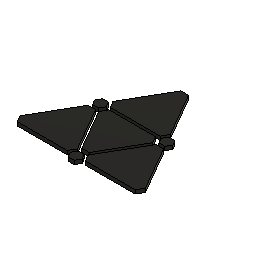
FumeExtractorFusionCAD (Autodesk Fusion 360 archive; units mm, degrees)
design "logoV2"
Autodesk Fusion 360 part; units mm, degrees
sketch "Sketch1" plane through (0, 0, 0) normal (0, 0, 1) x (1, 0, 0)
  line L0 (-18.1865, -0.75) -> (-35.507, -30.75)
  line L1 (-35.507, -30.75) -> (-0.866, -30.75)
  line L2 (-0.866, -30.75) -> (-18.1865, -0.75)
  line L3 (17.3205, 0.75) -> (0, 30.75)
  line L4 (-17.3205, 0.75) -> (17.3205, 0.75)
  line L5 (0, 30.75) -> (-17.3205, 0.75)
  line L6 (35.507, -30.75) -> (18.1865, -0.75)
  line L7 (0.866, -30.75) -> (35.507, -30.75)
  line L8 (18.1865, -0.75) -> (0.866, -30.75)
  line L9 (0, 10.75) -> (0, 0.75) construction
  line L10 (-17.3205, 0.75) -> (-18.1865, -0.75) construction
  line L11 (17.3205, 0.75) -> (18.1865, -0.75) construction
  line L12 (16.4545, -0.75) -> (0, -29.25)
  line L13 (-16.4545, -0.75) -> (16.4545, -0.75)
  line L14 (0, -29.25) -> (-16.4545, -0.75)
  point P0 (-18.1865, -20.75)
  point P1 (0, 10.75)
  point P2 (18.1865, -20.75)
  dimension "d2" = 10
  dimension "d3" = 10
  dimension "d4" = 10
  dimension "d6" = 34.641
  dimension "d8" = 20
  dimension "d9" = 20.75
  dimension "d11" = 0.75
  dimension "d16" = 1.5
  dimension "d17" = 1.5
  dimension "d18" = 1.5
  constraint horizontal L1
  constraint horizontal L4
  constraint horizontal L7
  constraint horizontal P0 P2
  constraint coincident P1 L9.start
  constraint vertical L9
  constraint coincident L4 L9.end
  constraint vertical origin L9.end
  constraint parallel L5 L10
  constraint coincident L0.start L2.end
  constraint parallel L3 L11
  constraint coincident L6.end L8.start
  constraint coincident L13.start L14.end
  constraint coincident L12.start L13.end
  constraint coincident L12.end L14.start
  measures "d2" distance of P0 L2
  measures "d3" distance of P1 L3
  measures "d4" distance of P2 L6
  measures "d6" distance of L0.end L1.end
  measures "d8" distance of L0.start P0
  measures "d9" vertical distance of origin P0
  measures "d11" distance of origin L9.end
extrude "Extrude1" add sketch "Sketch1" along normal blind 2 makes body 1 at (0, 10.75, 0) makes body 2 at (-18.1865, -20.75, 0) makes body 3 at (18.1865, -20.75, 0) makes body 4 at (0, -10.25, 0)
chamfer "Chamfer1" distance 4 angle 45 9 edges at (0.866, -30.75, 1) (35.507, -30.75, 1) (18.1865, -0.75, 1) (-0.866, -30.75, 1) (-35.507, -30.75, 1) (-18.1865, -0.75, 1) (17.3205, 0.75, 1) (0, 30.75, 1) (-17.3205, 0.75, 1) on bodies 1 2 3
chamfer "Chamfer2" distance 4 angle 45 3 edges at (0, -29.25, 1) (16.4545, -0.75, 1) (-16.4545, -0.75, 1) on bodies 4
sketch "Sketch2" plane through (0, 0, 2) normal (0, 0, 1) x (-1, 0, 0)
  line L0 (12.4545, 0.75) -> (14.4545, 4.2141)
  line L1 (14.4545, 4.2141) -> (2, 25.7859)
  line L2 (2, 25.7859) -> (-2, 25.7859)
  line L3 (-2, 25.7859) -> (-14.4545, 4.2141)
  line L4 (-14.4545, 4.2141) -> (-12.4545, 0.75)
  line L5 (-12.4545, 0.75) -> (12.4545, 0.75)
  line L6 (16.1865, 4.2141) -> (20.1865, 4.2141)
  line L7 (20.1865, 4.2141) -> (33.507, 27.2859)
  line L8 (33.507, 27.2859) -> (31.507, 30.75)
  line L9 (31.507, 30.75) -> (4.866, 30.75)
  line L10 (4.866, 30.75) -> (2.866, 27.2859)
  line L11 (2.866, 27.2859) -> (16.1865, 4.2141)
  line L12 (-20.1865, 4.2141) -> (-16.1865, 4.2141)
  line L13 (-16.1865, 4.2141) -> (-2.866, 27.2859)
  line L14 (-2.866, 27.2859) -> (-4.866, 30.75)
  line L15 (-4.866, 30.75) -> (-31.507, 30.75)
  line L16 (-31.507, 30.75) -> (-33.507, 27.2859)
  line L17 (-33.507, 27.2859) -> (-20.1865, 4.2141)
  line L18 (4.866, 30.75) -> (-4.866, 30.75)
  line L19 (2.433, 26.5359) -> (4.866, 30.75)
  line L20 (4.866, 30.75) -> (2.433, 34.9641)
  line L21 (2.433, 34.9641) -> (-2.433, 34.9641)
  line L22 (-2.433, 34.9641) -> (-4.866, 30.75)
  line L23 (-4.866, 30.75) -> (-2.433, 26.5359)
  line L24 (-2.433, 26.5359) -> (2.433, 26.5359)
  line L25 (1.567, 28.0359) -> (3.134, 30.75)
  line L26 (3.134, 30.75) -> (1.567, 33.4641)
  line L27 (1.567, 33.4641) -> (-1.567, 33.4641)
  line L28 (-1.567, 33.4641) -> (-3.134, 30.75)
  line L29 (-3.134, 30.75) -> (-1.567, 28.0359)
  line L30 (-1.567, 28.0359) -> (1.567, 28.0359)
  line L31 (0, 25.7859) -> (0, 0.75) construction
  line L32 (8.2272, 15) -> (-13.4545, 2.4821) construction
  line L33 (-8.2272, 15) -> (13.4545, 2.4821) construction
  point P0 (0, 30.75)
  point P1 (0, 30.75)
  point P2 (0, 10.25)
  dimension "d20" = 1.5
  constraint coincident L9.end L10.start
  constraint coincident L14.end L15.start
  constraint midpoint L18 P1
  constraint horizontal L24
  constraint coincident L10.end L19
  constraint coincident P1 P0
  constraint midpoint L2 L31.start
  constraint midpoint L5 L31.end
  constraint midpoint L1 L32.start
  constraint midpoint L4 L32.end
  constraint midpoint L3 L33.start
  constraint midpoint L0 L33.end
  constraint coincident L31 P2
  constraint coincident L33 P2
  measures "d20" distance of L24 L30
extrude "Extrude2" add sketch "Sketch2" against normal blind 2 separate body contours L18 L25 L29 L30 | L18 L26 L27 L28 makes body 5
pattern_circular "C-Pattern1" count 3 over 360 about axis through (0, -10.25, -128.8735) along (0, 0, 1) of "Extrude2" makes body 6 at (18.7982, 0, 2) makes body 7 at (-16.7089, 0, 2)
equation "scale = 1 mm"
equation "d2 = 10 * scale"
equation "d3 = d2"
equation "d4 = d2"
equation "d5 = d6 / 2 + spacing / 2"
equation "d9 = d8 + spacing / 2"
equation "spacing = 1.5 * scale"
equation "d11 = spacing / 2"
equation "d12 = height"
equation "d14 = chamfer"
equation "chamfer = 4 * scale"
equation "d16 = spacing"
equation "d17 = spacing"
equation "d18 = spacing"
equation "d19 = chamfer"
equation "d20 = spacing"
equation "d21 = -height"
equation "height = 2 mm"

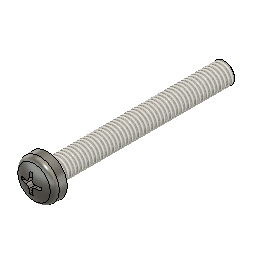
design "Pan Head Screw ISO 7045 - M3 x 25 - H Steel 4.6 Plain"
description: Pan Head Screw ISO 7045 - M3 x 25 - H
part number: ISO 7045 - M3 x 25 - H Steel 4.6 Plain
Autodesk Fusion 360 part; units mm, degrees
sketch "Sketch1" plane through (0, 0, 0) normal (0, 1, 0) x (1, 0, 0)
  line L0 (-1.5, 1) -> (-1.5, 25)
  line L1 (-1.5, 25) -> (0, 25)
  line L2 (0, 25) -> (0, -2.4)
  line L3 (-1.3647, 0) -> (-2.8, 0)
  arc A0 (-2.7449, -1.5792) -> (0, -2.4) centre (0, 2.6) ccw
  line L4 (-1.5, 1) -> (-1.3647, 0.7098)
  line L5 (-1.3647, 0.7098) -> (-1.3647, 0)
  line L6 (-2.8, 0) -> (-2.7449, -1.5792)
  dimension "d9" = 3
  dimension "d66" = 5.6
  dimension "d75" = 2.7294
  dimension "d77" = 1
  dimension "d78" = 155
  dimension "d103" = 2
  dimension "d111" = 2.4
  dimension "d112" = 25
  constraint perpendicular L0 L1
  constraint collinear origin L2.end L1.end
  constraint perpendicular L0 L3
  constraint coincident origin L3
  constraint vertical L0
  constraint vertical L2
  constraint coincident L2 A0.centre
  constraint perpendicular L3 L5
  constraint coincident L3.start L5.end
  measures "d77" distance of L3 L0.start
  measures "d78" angle of L0 L4
  measures "d103" angle of L2 L6
  measures "d111" distance of L2.end L3
  measures "d112" distance of origin L1
revolve "Revolve1" add sketch "Sketch1" angle 360 about axis through (0, 0, -25) along (0, 0, 1) makes body 1
ref_plane "WorkPlane1" through (0, 0, 2.4) normal (0, 0, 1) x (1, 0, 0)
sketch "Sketch2" plane through (0, 0, 2.4) normal (0, 0, 1) x (1, 0, 0)
  line L0 (-0.215, 0.215) -> (-1.5, 0.215)
  line L1 (-0.215, -0.215) -> (-1.5, -0.215)
  line L2 (-1.5, 0.215) -> (-1.5, -0.215)
  line L3 (-0.215, -0.215) -> (-0.215, -1.5)
  line L4 (-0.215, -1.5) -> (0.215, -1.5)
  line L5 (0.215, -0.215) -> (0.215, -1.5)
  line L6 (0.215, -0.215) -> (1.5, -0.215)
  line L7 (1.5, -0.215) -> (1.5, 0.215)
  line L8 (0.215, 0.215) -> (1.5, 0.215)
  line L9 (0.215, 0.215) -> (0.215, 1.5)
  line L10 (0.215, 1.5) -> (-0.215, 1.5)
  line L11 (-0.215, 0.215) -> (-0.215, 1.5)
  dimension "d105" = 0.43
  dimension "d107" = 360
  dimension "d108" = 3
  constraint perpendicular L1 L2
  constraint vertical L0.start L1.start
  constraint horizontal L1
  constraint coincident L8.start L9.start
  measures "d105" distance of L0 L1
  measures "d108" distance of L2 L7
extrude "Extrude1" add sketch "Sketch2" against normal blind 1.8 draft -4 separate body makes body 2
draft "Draft1" angle -30 neutral plane through (0, 0, 2.4) pull (0, 0, 1) 4 faces at (-1.458, -0.0297, 1.8) (0.0297, -1.458, 1.8) (1.458, 0.0297, 1.8) (-0.0297, 1.458, 1.8) on bodies 2
fillet "Fillet3" radius 0.43 4 edges at (0.1521, 0.1521, 1.5) (-0.1521, 0.1521, 1.5) (0.1521, -0.1521, 1.5) (-0.1521, -0.1521, 1.5) on bodies 2
combine "Combine1" operation cut target body 1 tool bodies 2
fillet "Fillet4" radius 0.9 1 edges at (-2.5591, 0.9926, 1.5792) on bodies 1
thread "Thread1" "ISO Metric profile 3.0 M3x0.5 M3x0.5 6g" major diameter 2.927 minor diameter 2.3555 pitch 0.5 angle 60 resizes the face on face at (-1.4981, 0.0748, -9) on bodies 1
fillet "Fillet5" radius 0.3 1 edges at (-1.2723, 0.4935, 0) on bodies 1
sketch "Sketch5" plane through (0, 0, 0) normal (0, 1, 0) x (1, 0, 0)
  line L0 (-1.53, 25) -> (-1.53, 24.6933)
  line L1 (-1.53, 24.6933) -> (-1.1933, 25)
  line L2 (0, 25) -> (0, -2.4)
  line L3 (-1.53, 25) -> (0, 25)
  dimension "d114" = 0.3067
  dimension "d115" = 1.53
  dimension "d116" = 0.3367
  constraint coincident L2.start L3.end
  constraint perpendicular L2 L3
  constraint coincident L1.end L3
  constraint perpendicular L0 L3
  measures "d114" distance of L0.end L3
  measures "d115" distance of L0 L2.start
  measures "d116" distance of L0 L1.end
revolve "Revolve2" cut sketch "Sketch5" angle 360 about axis through (0, 0, -25) along (0, 0, 1) bodies 1
equation "d9 = adsk_nomdia"
equation "adsk_nomlen = 25.00 mm"
equation "adsk_headh = 2.40 mm"
equation "adsk_headdia = 5.60 mm"
equation "adsk_nomdia = 3.00 mm"
equation "adsk_phildia = 3.00 mm"
equation "d31 = -adsk_phildepth"
equation "adsk_philwidth = 0.43 mm"
equation "adsk_phildepth = 1.80 mm"
equation "d66 = adsk_headdia"
equation "d71 = adsk_headh"
equation "adsk_thrlen = 24.00 mm"
equation "d75 = adsk_shnkdia"
equation "adsk_shnkdia = 2.72937 mm"
equation "d77 = adsk_nomlen - adsk_thrlen"
equation "adsk_endpointdia = 2.38655 mm"
equation "adsk_startlen = 0.306725 mm"
equation "adsk_ovalrad = 5.00 mm"
equation "adsk_headtoprad = adsk_nomdia * 0.3"
equation "adsk_midfillet = adsk_nomdia * 0.1"
equation "d98 = adsk_midfillet"
equation "adsk_headang = 2.00 deg"
equation "d102 = adsk_headtoprad"
equation "d103 = adsk_headang"
equation "d105 = adsk_philwidth"
equation "d108 = adsk_phildia"
equation "d110 = adsk_philwidth"
equation "d111 = adsk_headh"
equation "d112 = adsk_nomlen"
equation "d113 = ( adsk_nomlen + adsk_headh ) - ( adsk_ovalrad )"
equation "d114 = adsk_startlen"
equation "d115 = adsk_nomdia * 0.51"
equation "d116 = ( adsk_nomdia * 0.51 ) - ( adsk_endpointdia / 2 )"

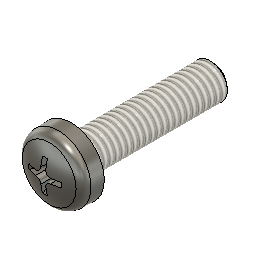
design "Pan Head Screw ISO 7045 - M3 x 12 - H Steel 4.6 Plain"
description: Pan Head Screw ISO 7045 - M3 x 12 - H
part number: ISO 7045 - M3 x 12 - H Steel 4.6 Plain
Autodesk Fusion 360 part; units mm, degrees
sketch "Sketch1" plane through (0, 0, 0) normal (0, 1, 0) x (1, 0, 0)
  line L0 (-1.5, 1) -> (-1.5, 12)
  line L1 (-1.5, 12) -> (0, 12)
  line L2 (0, 12) -> (0, -2.4)
  line L3 (-1.3647, 0) -> (-2.8, 0)
  arc A0 (-2.7449, -1.5792) -> (0, -2.4) centre (0, 2.6) ccw
  line L4 (-1.5, 1) -> (-1.3647, 0.7098)
  line L5 (-1.3647, 0.7098) -> (-1.3647, 0)
  line L6 (-2.8, 0) -> (-2.7449, -1.5792)
  dimension "d9" = 3
  dimension "d66" = 5.6
  dimension "d75" = 2.7294
  dimension "d77" = 1
  dimension "d78" = 155
  dimension "d103" = 2
  dimension "d111" = 2.4
  dimension "d112" = 12
  constraint perpendicular L0 L1
  constraint collinear origin L2.end L1.end
  constraint perpendicular L0 L3
  constraint coincident origin L3
  constraint vertical L0
  constraint vertical L2
  constraint coincident L2 A0.centre
  constraint perpendicular L3 L5
  constraint coincident L3.start L5.end
  measures "d77" distance of L3 L0.start
  measures "d78" angle of L0 L4
  measures "d103" angle of L2 L6
  measures "d111" distance of L2.end L3
  measures "d112" distance of origin L1
revolve "Revolve1" add sketch "Sketch1" angle 360 about axis through (0, 0, -12) along (0, 0, 1) makes body 1
ref_plane "WorkPlane1" through (0, 0, 2.4) normal (0, 0, 1) x (1, 0, 0)
sketch "Sketch2" plane through (0, 0, 2.4) normal (0, 0, 1) x (1, 0, 0)
  line L0 (-0.215, 0.215) -> (-1.5, 0.215)
  line L1 (-0.215, -0.215) -> (-1.5, -0.215)
  line L2 (-1.5, 0.215) -> (-1.5, -0.215)
  line L3 (-0.215, -0.215) -> (-0.215, -1.5)
  line L4 (-0.215, -1.5) -> (0.215, -1.5)
  line L5 (0.215, -0.215) -> (0.215, -1.5)
  line L6 (0.215, -0.215) -> (1.5, -0.215)
  line L7 (1.5, -0.215) -> (1.5, 0.215)
  line L8 (0.215, 0.215) -> (1.5, 0.215)
  line L9 (0.215, 0.215) -> (0.215, 1.5)
  line L10 (0.215, 1.5) -> (-0.215, 1.5)
  line L11 (-0.215, 0.215) -> (-0.215, 1.5)
  dimension "d105" = 0.43
  dimension "d107" = 360
  dimension "d108" = 3
  constraint perpendicular L1 L2
  constraint vertical L0.start L1.start
  constraint horizontal L1
  constraint coincident L8.start L9.start
  measures "d105" distance of L0 L1
  measures "d108" distance of L2 L7
extrude "Extrude1" add sketch "Sketch2" against normal blind 1.8 draft -4 separate body makes body 2
draft "Draft1" angle -30 neutral plane through (0, 0, 2.4) pull (0, 0, 1) 4 faces at (-1.458, 0.0297, 1.8) (-0.0297, -1.458, 1.8) (1.458, -0.0297, 1.8) (-0.0297, 1.458, 1.8) on bodies 2
fillet "Fillet3" radius 0.43 4 edges at (0.1521, 0.1521, 1.5) (-0.1521, 0.1521, 1.5) (0.1521, -0.1521, 1.5) (-0.1521, -0.1521, 1.5) on bodies 2
combine "Combine1" operation cut target body 1 tool bodies 2
fillet "Fillet4" radius 0.9 1 edges at (-2.5591, 0.9926, 1.5792) on bodies 1
thread "Thread1" "ISO Metric profile 3.0 M3x0.5 M3x0.5 6g" major diameter 2.927 minor diameter 2.3555 pitch 0.5 angle 60 resizes the face on face at (-1.4981, 0.0748, -4.6667) on bodies 1
fillet "Fillet5" radius 0.3 1 edges at (-1.2723, 0.4935, 0) on bodies 1
sketch "Sketch5" plane through (0, 0, 0) normal (0, 1, 0) x (1, 0, 0)
  line L0 (-1.53, 12) -> (-1.53, 11.6933)
  line L1 (-1.53, 11.6933) -> (-1.1933, 12)
  line L2 (0, 12) -> (0, -2.4)
  line L3 (-1.53, 12) -> (0, 12)
  dimension "d114" = 0.3067
  dimension "d115" = 1.53
  dimension "d116" = 0.3367
  constraint coincident L2.start L3.end
  constraint perpendicular L2 L3
  constraint coincident L1.end L3
  constraint perpendicular L0 L3
  measures "d114" distance of L0.end L3
  measures "d115" distance of L0 L2.start
  measures "d116" distance of L0 L1.end
revolve "Revolve2" cut sketch "Sketch5" angle 360 about axis through (0, 0, -12) along (0, 0, 1) bodies 1
equation "d9 = adsk_nomdia"
equation "adsk_nomlen = 12.00 mm"
equation "adsk_headh = 2.40 mm"
equation "adsk_headdia = 5.60 mm"
equation "adsk_nomdia = 3.00 mm"
equation "adsk_phildia = 3.00 mm"
equation "d31 = -adsk_phildepth"
equation "adsk_philwidth = 0.43 mm"
equation "adsk_phildepth = 1.80 mm"
equation "d66 = adsk_headdia"
equation "d71 = adsk_headh"
equation "adsk_thrlen = 11.00 mm"
equation "d75 = adsk_shnkdia"
equation "adsk_shnkdia = 2.72937 mm"
equation "d77 = adsk_nomlen - adsk_thrlen"
equation "adsk_endpointdia = 2.38655 mm"
equation "adsk_startlen = 0.306725 mm"
equation "adsk_ovalrad = 5.00 mm"
equation "adsk_headtoprad = adsk_nomdia * 0.3"
equation "adsk_midfillet = adsk_nomdia * 0.1"
equation "d98 = adsk_midfillet"
equation "adsk_headang = 2.00 deg"
equation "d102 = adsk_headtoprad"
equation "d103 = adsk_headang"
equation "d105 = adsk_philwidth"
equation "d108 = adsk_phildia"
equation "d110 = adsk_philwidth"
equation "d111 = adsk_headh"
equation "d112 = adsk_nomlen"
equation "d113 = ( adsk_nomlen + adsk_headh ) - ( adsk_ovalrad )"
equation "d114 = adsk_startlen"
equation "d115 = adsk_nomdia * 0.51"
equation "d116 = ( adsk_nomdia * 0.51 ) - ( adsk_endpointdia / 2 )"

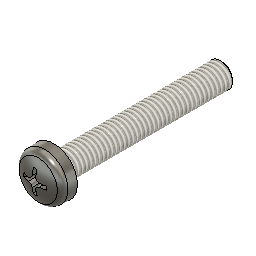
design "Pan Head Screw ISO 7045 - M3 x 20 - H Steel 4.6 Plain"
description: Pan Head Screw ISO 7045 - M3 x 20 - H
part number: ISO 7045 - M3 x 20 - H Steel 4.6 Plain
Autodesk Fusion 360 part; units mm, degrees
sketch "Sketch1" plane through (0, 0, 0) normal (0, 1, 0) x (1, 0, 0)
  line L0 (-1.5, 1) -> (-1.5, 20)
  line L1 (-1.5, 20) -> (0, 20)
  line L2 (0, 20) -> (0, -2.4)
  line L3 (-1.3647, 0) -> (-2.8, 0)
  arc A0 (-2.7449, -1.5792) -> (0, -2.4) centre (0, 2.6) ccw
  line L4 (-1.5, 1) -> (-1.3647, 0.7098)
  line L5 (-1.3647, 0.7098) -> (-1.3647, 0)
  line L6 (-2.8, 0) -> (-2.7449, -1.5792)
  dimension "d9" = 3
  dimension "d66" = 5.6
  dimension "d75" = 2.7294
  dimension "d77" = 1
  dimension "d78" = 155
  dimension "d103" = 2
  dimension "d111" = 2.4
  dimension "d112" = 20
  constraint perpendicular L0 L1
  constraint collinear origin L2.end L1.end
  constraint perpendicular L0 L3
  constraint coincident origin L3
  constraint vertical L0
  constraint vertical L2
  constraint coincident L2 A0.centre
  constraint perpendicular L3 L5
  constraint coincident L3.start L5.end
  measures "d77" distance of L3 L0.start
  measures "d78" angle of L0 L4
  measures "d103" angle of L2 L6
  measures "d111" distance of L2.end L3
  measures "d112" distance of origin L1
revolve "Revolve1" add sketch "Sketch1" angle 360 about axis through (0, 0, -20) along (0, 0, 1) makes body 1
ref_plane "WorkPlane1" through (0, 0, 2.4) normal (0, 0, 1) x (1, 0, 0)
sketch "Sketch2" plane through (0, 0, 2.4) normal (0, 0, 1) x (1, 0, 0)
  line L0 (-0.215, 0.215) -> (-1.5, 0.215)
  line L1 (-0.215, -0.215) -> (-1.5, -0.215)
  line L2 (-1.5, 0.215) -> (-1.5, -0.215)
  line L3 (-0.215, -0.215) -> (-0.215, -1.5)
  line L4 (-0.215, -1.5) -> (0.215, -1.5)
  line L5 (0.215, -0.215) -> (0.215, -1.5)
  line L6 (0.215, -0.215) -> (1.5, -0.215)
  line L7 (1.5, -0.215) -> (1.5, 0.215)
  line L8 (0.215, 0.215) -> (1.5, 0.215)
  line L9 (0.215, 0.215) -> (0.215, 1.5)
  line L10 (0.215, 1.5) -> (-0.215, 1.5)
  line L11 (-0.215, 0.215) -> (-0.215, 1.5)
  dimension "d105" = 0.43
  dimension "d107" = 360
  dimension "d108" = 3
  constraint perpendicular L1 L2
  constraint vertical L0.start L1.start
  constraint horizontal L1
  constraint coincident L8.start L9.start
  measures "d105" distance of L0 L1
  measures "d108" distance of L2 L7
extrude "Extrude1" add sketch "Sketch2" against normal blind 1.8 draft -4 separate body makes body 2
draft "Draft1" angle -30 neutral plane through (0, 0, 2.4) pull (0, 0, 1) 4 faces at (-1.458, -0.0297, 1.8) (0.0297, -1.458, 1.8) (1.458, 0.0297, 1.8) (-0.0297, 1.458, 1.8) on bodies 2
fillet "Fillet3" radius 0.43 4 edges at (0.1521, 0.1521, 1.5) (-0.1521, 0.1521, 1.5) (0.1521, -0.1521, 1.5) (-0.1521, -0.1521, 1.5) on bodies 2
combine "Combine1" operation cut target body 1 tool bodies 2
fillet "Fillet4" radius 0.9 1 edges at (-2.5591, 0.9926, 1.5792) on bodies 1
thread "Thread1" "ISO Metric profile 3.0 M3x0.5 M3x0.5 6g" major diameter 2.927 minor diameter 2.3555 pitch 0.5 angle 60 resizes the face on face at (-1.4981, 0.0748, -13.6667) on bodies 1
fillet "Fillet5" radius 0.3 1 edges at (-1.2723, 0.4935, 0) on bodies 1
sketch "Sketch5" plane through (0, 0, 0) normal (0, 1, 0) x (1, 0, 0)
  line L0 (-1.53, 20) -> (-1.53, 19.6933)
  line L1 (-1.53, 19.6933) -> (-1.1933, 20)
  line L2 (0, 20) -> (0, -2.4)
  line L3 (-1.53, 20) -> (0, 20)
  dimension "d114" = 0.3067
  dimension "d115" = 1.53
  dimension "d116" = 0.3367
  constraint coincident L2.start L3.end
  constraint perpendicular L2 L3
  constraint coincident L1.end L3
  constraint perpendicular L0 L3
  measures "d114" distance of L0.end L3
  measures "d115" distance of L0 L2.start
  measures "d116" distance of L0 L1.end
revolve "Revolve2" cut sketch "Sketch5" angle 360 about axis through (0, 0, -20) along (0, 0, 1) bodies 1
equation "d9 = adsk_nomdia"
equation "adsk_nomlen = 20.00 mm"
equation "adsk_headh = 2.40 mm"
equation "adsk_headdia = 5.60 mm"
equation "adsk_nomdia = 3.00 mm"
equation "adsk_phildia = 3.00 mm"
equation "d31 = -adsk_phildepth"
equation "adsk_philwidth = 0.43 mm"
equation "adsk_phildepth = 1.80 mm"
equation "d66 = adsk_headdia"
equation "d71 = adsk_headh"
equation "adsk_thrlen = 19.00 mm"
equation "d75 = adsk_shnkdia"
equation "adsk_shnkdia = 2.72937 mm"
equation "d77 = adsk_nomlen - adsk_thrlen"
equation "adsk_endpointdia = 2.38655 mm"
equation "adsk_startlen = 0.306725 mm"
equation "adsk_ovalrad = 5.00 mm"
equation "adsk_headtoprad = adsk_nomdia * 0.3"
equation "adsk_midfillet = adsk_nomdia * 0.1"
equation "d98 = adsk_midfillet"
equation "adsk_headang = 2.00 deg"
equation "d102 = adsk_headtoprad"
equation "d103 = adsk_headang"
equation "d105 = adsk_philwidth"
equation "d108 = adsk_phildia"
equation "d110 = adsk_philwidth"
equation "d111 = adsk_headh"
equation "d112 = adsk_nomlen"
equation "d113 = ( adsk_nomlen + adsk_headh ) - ( adsk_ovalrad )"
equation "d114 = adsk_startlen"
equation "d115 = adsk_nomdia * 0.51"
equation "d116 = ( adsk_nomdia * 0.51 ) - ( adsk_endpointdia / 2 )"

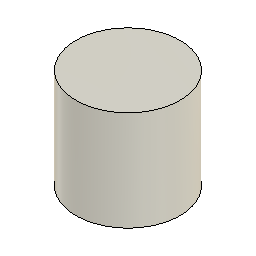
design "fanPlaceholderV1"
Autodesk Fusion 360 part; units mm, degrees
sketch "Sketch1" plane through (0, 0, 0) normal (0, 0, 1) x (1, 0, 0)
  circle A0 centre (0, 0) radius 50
  dimension "d1" = 100
  constraint coincident A0.centre origin
  measures "d1" diameter of A0
extrude "Extrude1" add sketch "Sketch1" along normal blind 96

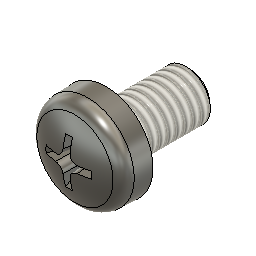
design "Pan Head Screw ISO 7045 - M3 x 5 - H Steel 4.6 Plain"
description: Pan Head Screw ISO 7045 - M3 x 5 - H
part number: ISO 7045 - M3 x 5 - H Steel 4.6 Plain
Autodesk Fusion 360 part; units mm, degrees
sketch "Sketch1" plane through (0, 0, 0) normal (0, 1, 0) x (1, 0, 0)
  line L0 (-1.5, 1) -> (-1.5, 5)
  line L1 (-1.5, 5) -> (0, 5)
  line L2 (0, 5) -> (0, -2.4)
  line L3 (-1.3647, 0) -> (-2.8, 0)
  arc A0 (-2.7449, -1.5792) -> (0, -2.4) centre (0, 2.6) ccw
  line L4 (-1.5, 1) -> (-1.3647, 0.7098)
  line L5 (-1.3647, 0.7098) -> (-1.3647, 0)
  line L6 (-2.8, 0) -> (-2.7449, -1.5792)
  dimension "d9" = 3
  dimension "d66" = 5.6
  dimension "d75" = 2.7294
  dimension "d77" = 1
  dimension "d78" = 155
  dimension "d103" = 2
  dimension "d111" = 2.4
  dimension "d112" = 5
  constraint perpendicular L0 L1
  constraint collinear origin L2.end L1.end
  constraint perpendicular L0 L3
  constraint coincident origin L3
  constraint vertical L0
  constraint vertical L2
  constraint coincident L2 A0.centre
  constraint perpendicular L3 L5
  constraint coincident L3.start L5.end
  measures "d77" distance of L3 L0.start
  measures "d78" angle of L0 L4
  measures "d103" angle of L2 L6
  measures "d111" distance of L2.end L3
  measures "d112" distance of origin L1
revolve "Revolve1" add sketch "Sketch1" angle 360 about axis through (0, 0, -5) along (0, 0, 1) makes body 1
ref_plane "WorkPlane1" through (0, 0, 2.4) normal (0, 0, 1) x (1, 0, 0)
sketch "Sketch2" plane through (0, 0, 2.4) normal (0, 0, 1) x (1, 0, 0)
  line L0 (-0.215, 0.215) -> (-1.5, 0.215)
  line L1 (-0.215, -0.215) -> (-1.5, -0.215)
  line L2 (-1.5, 0.215) -> (-1.5, -0.215)
  line L3 (-0.215, -0.215) -> (-0.215, -1.5)
  line L4 (-0.215, -1.5) -> (0.215, -1.5)
  line L5 (0.215, -0.215) -> (0.215, -1.5)
  line L6 (0.215, -0.215) -> (1.5, -0.215)
  line L7 (1.5, -0.215) -> (1.5, 0.215)
  line L8 (0.215, 0.215) -> (1.5, 0.215)
  line L9 (0.215, 0.215) -> (0.215, 1.5)
  line L10 (0.215, 1.5) -> (-0.215, 1.5)
  line L11 (-0.215, 0.215) -> (-0.215, 1.5)
  dimension "d105" = 0.43
  dimension "d107" = 360
  dimension "d108" = 3
  constraint perpendicular L1 L2
  constraint vertical L0.start L1.start
  constraint horizontal L1
  constraint coincident L8.start L9.start
  measures "d105" distance of L0 L1
  measures "d108" distance of L2 L7
extrude "Extrude1" add sketch "Sketch2" against normal blind 1.8 draft -4 separate body makes body 2
draft "Draft1" angle -30 neutral plane through (0, 0, 2.4) pull (0, 0, 1) 4 faces at (-1.458, 0.0297, 1.8) (0.0297, -1.458, 1.8) (1.458, -0.0297, 1.8) (0.0297, 1.458, 1.8) on bodies 2
fillet "Fillet3" radius 0.43 4 edges at (0.1521, 0.1521, 1.5) (-0.1521, 0.1521, 1.5) (0.1521, -0.1521, 1.5) (-0.1521, -0.1521, 1.5) on bodies 2
combine "Combine1" operation cut target body 1 tool bodies 2
fillet "Fillet4" radius 0.9 1 edges at (-2.5591, 0.9926, 1.5792) on bodies 1
thread "Thread1" "ISO Metric profile 3.0 M3x0.5 M3x0.5 6g" major diameter 2.927 minor diameter 2.3555 pitch 0.5 angle 60 resizes the face on face at (-1.4981, 0.0748, -2.3333) on bodies 1
fillet "Fillet5" radius 0.3 1 edges at (-1.2723, 0.4935, 0) on bodies 1
sketch "Sketch5" plane through (0, 0, 0) normal (0, 1, 0) x (1, 0, 0)
  line L0 (-1.53, 5) -> (-1.53, 4.6933)
  line L1 (-1.53, 4.6933) -> (-1.1933, 5)
  line L2 (0, 5) -> (0, -2.4)
  line L3 (-1.53, 5) -> (0, 5)
  dimension "d114" = 0.3067
  dimension "d115" = 1.53
  dimension "d116" = 0.3367
  constraint coincident L2.start L3.end
  constraint perpendicular L2 L3
  constraint coincident L1.end L3
  constraint perpendicular L0 L3
  measures "d114" distance of L0.end L3
  measures "d115" distance of L0 L2.start
  measures "d116" distance of L0 L1.end
revolve "Revolve2" cut sketch "Sketch5" angle 360 about axis through (0, 0, -5) along (0, 0, 1) bodies 1
equation "d9 = adsk_nomdia"
equation "adsk_nomlen = 5.00 mm"
equation "adsk_headh = 2.40 mm"
equation "adsk_headdia = 5.60 mm"
equation "adsk_nomdia = 3.00 mm"
equation "adsk_phildia = 3.00 mm"
equation "d31 = -adsk_phildepth"
equation "adsk_philwidth = 0.43 mm"
equation "adsk_phildepth = 1.80 mm"
equation "d66 = adsk_headdia"
equation "d71 = adsk_headh"
equation "adsk_thrlen = 4.00 mm"
equation "d75 = adsk_shnkdia"
equation "adsk_shnkdia = 2.72937 mm"
equation "d77 = adsk_nomlen - adsk_thrlen"
equation "adsk_endpointdia = 2.38655 mm"
equation "adsk_startlen = 0.306725 mm"
equation "adsk_ovalrad = 5.00 mm"
equation "adsk_headtoprad = adsk_nomdia * 0.3"
equation "adsk_midfillet = adsk_nomdia * 0.1"
equation "d98 = adsk_midfillet"
equation "adsk_headang = 2.00 deg"
equation "d102 = adsk_headtoprad"
equation "d103 = adsk_headang"
equation "d105 = adsk_philwidth"
equation "d108 = adsk_phildia"
equation "d110 = adsk_philwidth"
equation "d111 = adsk_headh"
equation "d112 = adsk_nomlen"
equation "d113 = ( adsk_nomlen + adsk_headh ) - ( adsk_ovalrad )"
equation "d114 = adsk_startlen"
equation "d115 = adsk_nomdia * 0.51"
equation "d116 = ( adsk_nomdia * 0.51 ) - ( adsk_endpointdia / 2 )"

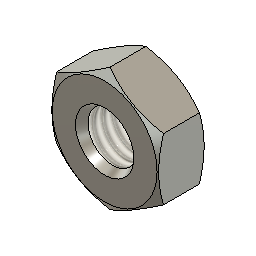
design "Hexagon Regular Nut ISO 4032 - M3 Steel 6 Plain"
description: Hexagon Regular Nut ISO 4032 - M3
part number: ISO 4032 - M3 Steel 6 Plain
Autodesk Fusion 360 part; units mm, degrees
sketch "Sketch1" plane through (0, 0, 0) normal (0, 1, 0) x (1, 0, 0)
  line L0 (0, 0) -> (0, -2.4)
  line L1 (-1.5, 0) -> (-2.695, 0)
  line L2 (-2.695, 0) -> (-3.1763, -0.2778)
  line L3 (-3.1763, -0.2778) -> (-3.1763, -2.1222)
  line L4 (-3.1763, -2.1222) -> (-2.695, -2.4)
  line L5 (-2.695, -2.4) -> (-1.5, -2.4)
  line L6 (-1.5, -2.4) -> (-1.5, 0)
  dimension "d121" = 3
  dimension "d122" = 30
  dimension "d123" = 30
  dimension "d128" = 6.3525
  dimension "d172" = 5.39
  dimension "d179" = 2.4
  constraint vertical L0
  constraint coincident L0 L0.end
  constraint coincident origin L0
  constraint horizontal L1
  constraint coincident L0.start L1
  constraint coincident L0.start origin
  constraint coincident L0.end L5
  constraint vertical L1.end L4.end
  measures "d122" angle of L1 L2
  measures "d123" angle of L4 L5
  measures "d179" distance of L1 L5
revolve "Revolve1" add sketch "Sketch1" angle 360 about axis through (0, 0, 0) along (0, 0, 1)
sketch "Sketch8" plane through (0, 0, 2.4) normal (0, 0, 1) x (1, 0, 0)
  line L0 (-2.75, -1.5894) -> (-2.75, 1.5894)
  circle A0 centre (0, 0) radius 1.5
  circle A1 centre (0, 0) radius 3.1763
  dimension "d114" = 2.75
  constraint coincident L0.end A1
  constraint coincident L0.start A1
  constraint vertical L0
  measures "d114" distance of A0.centre L0
extrude "Extrude5" cut sketch "Sketch8" against normal blind 2.4 contours L0 A1 picked at (-2.8188, -0.3871)
pattern_circular "C-Pattern2" count 6 over 360 about axis through (0, 0, 1.75) along (0, 0, 1) of "Extrude5"
thread "Thread3" "ISO Metric profile 3.0 M3x0.5 M3x0.5 6H" major diameter 3.086 minor diameter 2.529 pitch 0.5 angle 60 resizes the face on face at (-1.4925, 0.1494, 1.6)
sketch "Sketch12" plane through (0, 0, 0) normal (0, 1, 0) x (1, 0, 0)
  line L0 (-1.5, 0) -> (0, 0)
  line L1 (-0.8072, -1.2) -> (-1.5, 0)
  line L2 (-1.5, -2.4) -> (0, -2.4)
  line L3 (-0.8072, -1.2) -> (-1.5, -2.4)
  line L4 (0, 0) -> (0, -2.4)
  dimension "d169" = 60
  dimension "d177" = 1.5
  dimension "d178" = 60
  constraint horizontal L0
  constraint coincident L1.start L3.start
  constraint vertical L0.start L2.start
  constraint coincident L2.end L4.end
  constraint coincident L0.end L4.start
  constraint perpendicular L2 L4
  measures "d169" angle of L2 L3
  measures "d177" distance of L0.start L4
  measures "d178" angle of L0 L1
revolve "Revolve3" cut sketch "Sketch12" angle 360 about axis through (0, 0, 1.75) along (0, 0, 1)
equation "adsk_nheig = 2.40 mm"
equation "adsk_maxdia = 6.3525 mm"
equation "adsk_nomdia = 3.00 mm"
equation "d89 = -adsk_nheig"
equation "adsk_waflat = 5.50 mm"
equation "d114 = adsk_waflat / 2"
equation "adsk_chamang1 = 30.00 deg"
equation "adsk_chamang2 = 30.00 deg"
equation "d121 = adsk_nomdia"
equation "d122 = adsk_chamang1"
equation "d123 = adsk_chamang2"
equation "d128 = adsk_maxdia"
equation "d163 = adsk_nheig"
equation "adsk_beardia = 5.39 mm"
equation "d172 = adsk_beardia"
equation "d177 = adsk_nomdia * 0.5"
equation "d179 = adsk_nheig"

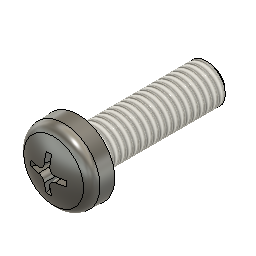
design "Pan Head Screw ISO 7045 - M3 x 10 - H Steel 4.6 Plain"
description: Pan Head Screw ISO 7045 - M3 x 10 - H
part number: ISO 7045 - M3 x 10 - H Steel 4.6 Plain
Autodesk Fusion 360 part; units mm, degrees
sketch "Sketch1" plane through (0, 0, 0) normal (0, 1, 0) x (1, 0, 0)
  line L0 (-1.5, 1) -> (-1.5, 10)
  line L1 (-1.5, 10) -> (0, 10)
  line L2 (0, 10) -> (0, -2.4)
  line L3 (-1.3647, 0) -> (-2.8, 0)
  arc A0 (-2.7449, -1.5792) -> (0, -2.4) centre (0, 2.6) ccw
  line L4 (-1.5, 1) -> (-1.3647, 0.7098)
  line L5 (-1.3647, 0.7098) -> (-1.3647, 0)
  line L6 (-2.8, 0) -> (-2.7449, -1.5792)
  dimension "d9" = 3
  dimension "d66" = 5.6
  dimension "d75" = 2.7294
  dimension "d77" = 1
  dimension "d78" = 155
  dimension "d103" = 2
  dimension "d111" = 2.4
  dimension "d112" = 10
  constraint perpendicular L0 L1
  constraint collinear origin L2.end L1.end
  constraint perpendicular L0 L3
  constraint coincident origin L3
  constraint vertical L0
  constraint vertical L2
  constraint coincident L2 A0.centre
  constraint perpendicular L3 L5
  constraint coincident L3.start L5.end
  measures "d77" distance of L3 L0.start
  measures "d78" angle of L0 L4
  measures "d103" angle of L2 L6
  measures "d111" distance of L2.end L3
  measures "d112" distance of origin L1
revolve "Revolve1" add sketch "Sketch1" angle 360 about axis through (0, 0, -10) along (0, 0, 1) makes body 1
ref_plane "WorkPlane1" through (0, 0, 2.4) normal (0, 0, 1) x (1, 0, 0)
sketch "Sketch2" plane through (0, 0, 2.4) normal (0, 0, 1) x (1, 0, 0)
  line L0 (-0.215, 0.215) -> (-1.5, 0.215)
  line L1 (-0.215, -0.215) -> (-1.5, -0.215)
  line L2 (-1.5, 0.215) -> (-1.5, -0.215)
  line L3 (-0.215, -0.215) -> (-0.215, -1.5)
  line L4 (-0.215, -1.5) -> (0.215, -1.5)
  line L5 (0.215, -0.215) -> (0.215, -1.5)
  line L6 (0.215, -0.215) -> (1.5, -0.215)
  line L7 (1.5, -0.215) -> (1.5, 0.215)
  line L8 (0.215, 0.215) -> (1.5, 0.215)
  line L9 (0.215, 0.215) -> (0.215, 1.5)
  line L10 (0.215, 1.5) -> (-0.215, 1.5)
  line L11 (-0.215, 0.215) -> (-0.215, 1.5)
  dimension "d105" = 0.43
  dimension "d107" = 360
  dimension "d108" = 3
  constraint perpendicular L1 L2
  constraint vertical L0.start L1.start
  constraint horizontal L1
  constraint coincident L8.start L9.start
  measures "d105" distance of L0 L1
  measures "d108" distance of L2 L7
extrude "Extrude1" add sketch "Sketch2" against normal blind 1.8 draft -4 separate body makes body 2
draft "Draft1" angle -30 neutral plane through (0, 0, 2.4) pull (0, 0, 1) 4 faces at (-1.458, -0.0297, 1.8) (0.0297, -1.458, 1.8) (1.458, -0.0297, 1.8) (0.0297, 1.458, 1.8) on bodies 2
fillet "Fillet3" radius 0.43 4 edges at (0.1521, 0.1521, 1.5) (-0.1521, 0.1521, 1.5) (0.1521, -0.1521, 1.5) (-0.1521, -0.1521, 1.5) on bodies 2
combine "Combine1" operation cut target body 1 tool bodies 2
fillet "Fillet4" radius 0.9 1 edges at (-2.5591, 0.9926, 1.5792) on bodies 1
thread "Thread1" "ISO Metric profile 3.0 M3x0.5 M3x0.5 6g" major diameter 2.927 minor diameter 2.3555 pitch 0.5 angle 60 resizes the face on face at (-1.4925, 0.1494, -7) on bodies 1
fillet "Fillet5" radius 0.3 1 edges at (-1.2723, 0.4935, 0) on bodies 1
sketch "Sketch5" plane through (0, 0, 0) normal (0, 1, 0) x (1, 0, 0)
  line L0 (-1.53, 10) -> (-1.53, 9.6933)
  line L1 (-1.53, 9.6933) -> (-1.1933, 10)
  line L2 (0, 10) -> (0, -2.4)
  line L3 (-1.53, 10) -> (0, 10)
  dimension "d114" = 0.3067
  dimension "d115" = 1.53
  dimension "d116" = 0.3367
  constraint coincident L2.start L3.end
  constraint perpendicular L2 L3
  constraint coincident L1.end L3
  constraint perpendicular L0 L3
  measures "d114" distance of L0.end L3
  measures "d115" distance of L0 L2.start
  measures "d116" distance of L0 L1.end
revolve "Revolve2" cut sketch "Sketch5" angle 360 about axis through (0, 0, -10) along (0, 0, 1) bodies 1
equation "d9 = adsk_nomdia"
equation "adsk_nomlen = 10.00 mm"
equation "adsk_headh = 2.40 mm"
equation "adsk_headdia = 5.60 mm"
equation "adsk_nomdia = 3.00 mm"
equation "adsk_phildia = 3.00 mm"
equation "d31 = -adsk_phildepth"
equation "adsk_philwidth = 0.43 mm"
equation "adsk_phildepth = 1.80 mm"
equation "d66 = adsk_headdia"
equation "d71 = adsk_headh"
equation "adsk_thrlen = 9.00 mm"
equation "d75 = adsk_shnkdia"
equation "adsk_shnkdia = 2.72937 mm"
equation "d77 = adsk_nomlen - adsk_thrlen"
equation "adsk_endpointdia = 2.38655 mm"
equation "adsk_startlen = 0.306725 mm"
equation "adsk_ovalrad = 5.00 mm"
equation "adsk_headtoprad = adsk_nomdia * 0.3"
equation "adsk_midfillet = adsk_nomdia * 0.1"
equation "d98 = adsk_midfillet"
equation "adsk_headang = 2.00 deg"
equation "d102 = adsk_headtoprad"
equation "d103 = adsk_headang"
equation "d105 = adsk_philwidth"
equation "d108 = adsk_phildia"
equation "d110 = adsk_philwidth"
equation "d111 = adsk_headh"
equation "d112 = adsk_nomlen"
equation "d113 = ( adsk_nomlen + adsk_headh ) - ( adsk_ovalrad )"
equation "d114 = adsk_startlen"
equation "d115 = adsk_nomdia * 0.51"
equation "d116 = ( adsk_nomdia * 0.51 ) - ( adsk_endpointdia / 2 )"
